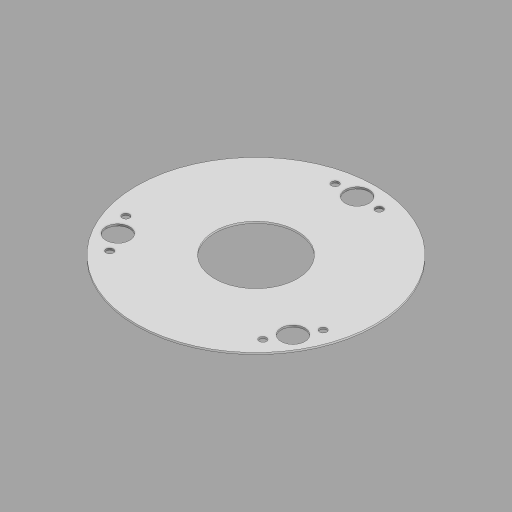
# Autodesk Inventor part: Baffle
Saved by Autodesk Inventor 2024 (Build 280153020, 153B)
## iProperties
Created: 2023-10-26
Part Number: Baffle
Material: Generic
Document SubType Name: Modeling
Designer: schanen
Density: 1 g/cm^3
Appearance: Default
Mass: 11.1966 g
Surface Area: 231.347 cm^2
Volume: 11.1966 cm^3
Author: schanen
Autodesk Inventor part; units mm, degrees
ref_plane "YZ Plane" through (0, 0, 0) normal (1, 0, 0) x (0, 1, 0)
ref_plane "XZ Plane" through (0, 0, 0) normal (0, 1, 0) x (-1, 0, 0)
ref_plane "XY Plane" through (0, 0, 0) normal (0, 0, 1) x (1, 0, 0)
sketch "Sketch1" plane through (0, 0, 0) normal (0, 0, 1) x (1, 0, 0)
  line L0 (0, 0) -> (-65, 0)
  line L1 (-65, 0) -> (-65, 1)
  line L2 (-65, 1) -> (0, 1)
  line L3 (0, 1) -> (0, 0)
  dimension "d0" = 65
  dimension "d1" = 1
  constraints: 8 end point, 2 parallel, 1 horizontal, 1 perpendicular
  measures "d0" distance of L1.end L2.end
  measures "d1" distance of L0.end L1.end
revolve "Revolution1" add sketch "Sketch1" angle 360 about axis through (0, 1, 0) along (0, -1, 0)
sketch "Sketch2" plane through (0, 1, 0) normal (0, 1, 0) x (1, 0, 0)
  circle A0 centre (0, 0) radius 22.5
  dimension "d3" = 45
  constraints: 1 centre point, 1 coincident
  measures "d3" diameter of A0
extrude "Extrusion1" cut sketch "Sketch2" against normal through all
sketch "Sketch3" plane through (0, 1, 0) normal (0, 1, 0) x (1, 0, 0)
  circle A0 centre (0, 55) radius 6.5
  circle A1 centre (-12, 55) radius 2
  circle A2 centre (12, 55) radius 2
  point P0 (0, 0)
  dimension "d12" = 13
  dimension "d13" = 55
  dimension "d14" = 4
  dimension "d15" = 12
  dimension "d16" = 4
  dimension "d17" = 12
  constraints: 3 centre point, 2 horizontal alignment, 1 vertical alignment
  measures "d12" diameter of A0
  measures "d13" distance of point (0, 0) A0.centre
  measures "d14" diameter of A1
  measures "d15" distance of A1.centre A0.centre
  measures "d16" diameter of A2
  measures "d17" distance of A2.centre A0.centre
extrude "Extrusion2" cut sketch "Sketch3" against normal through all
pattern_circular "Circular Pattern1" count 3 over 360 about axis through (0, 1, 0) along (0, -1, 0) of "Extrusion2"
equation "\"d17\" = d15"
body "Solid1"
